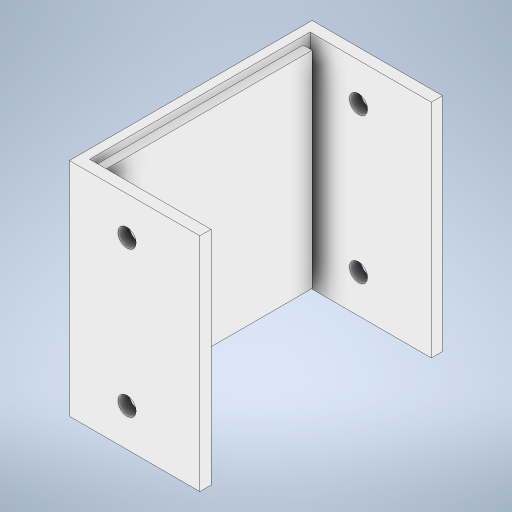
# Autodesk Inventor part: Tapa_R
Saved by Autodesk Inventor 2024 (Build 280153000, 153)
## iProperties
Created: 2023-05-26
Part Number: Tapa_R
Material: Plástico ABS
Document SubType Name: Modeling
Designer: epm01
Density: 1.06 g/cm^3
Appearance: Suave - Blanco
Mass: 7.0225 g
Surface Area: 64.215 cm^2
Volume: 6.625 cm^3
Author: epm01
Autodesk Inventor part; units mm, degrees
ref_plane "YZ Plane" through (0, 0, 0) normal (1, 0, 0) x (0, 1, 0)
ref_plane "XZ Plane" through (0, 0, 0) normal (0, 1, 0) x (-1, 0, 0)
ref_plane "XY Plane" through (0, 0, 0) normal (0, 0, 1) x (1, 0, 0)
sketch "Boceto1" plane through (0, 0, 0) normal (1, 0, 0) x (0, 1, 0)
  line L0 (-17, 17) -> (17, 17)
  line L1 (17, 17) -> (17, -17)
  line L2 (17, -17) -> (-17, -17)
  line L3 (-17, -17) -> (-17, 17)
  line L4 (-17, 17) -> (17, -17) construction
  line L5 (17, 17) -> (-17, -17) construction
  point P0 (0, 0)
  dimension "d0" = 34
  dimension "d1" = 34
  constraints: 12 end point, 2 midpoint, 2 parallel, 1 horizontal, 1 perpendicular
  measures "d0" distance of L0.end L1.end
  measures "d1" distance of L0.start L0.end
extrude "Extrusión1" add sketch "Boceto1" along normal blind 1.5
sketch "Boceto2" plane through (0, 0, 0) normal (-1, 0, 0) x (0, 0, 1)
  line L0 (-20, -18.25) -> (20, -18.25)
  line L1 (20, -18.25) -> (20, 18.25)
  line L2 (20, 18.25) -> (-20, 18.25)
  line L3 (-20, 18.25) -> (-20, -18.25)
  line L4 (-20, -18.25) -> (20, 18.25) construction
  line L5 (20, -18.25) -> (-20, 18.25) construction
  point P0 (0, 0)
  dimension "d4" = 36.5
  dimension "d5" = 40
  constraints: 12 end point, 2 midpoint, 2 parallel, 1 horizontal, 1 perpendicular
  measures "d4" distance of L0.end L1.end
  measures "d5" distance of L1.end L2.end
extrude "Extrusión2" add sketch "Boceto2" along normal blind 1.5
sketch "Boceto3" plane through (0, 0, 0) normal (1, 0, 0) x (0, 0, -1)
  line L0 (-20, 17.8927) -> (-20, -18.25)
  line L1 (-20, 18.25) -> (-20, -18.25)
  line L2 (20, -18.25) -> (-20, -18.25) projected
  line L3 (-18.15, -18.25) -> (-18.15, 18.25)
  line L4 (-18.15, 18.25) -> (-20, 18.25)
  line L5 (-20, -18.25) -> (-18.15, -18.25)
  line L6 (0, 18.25) -> (0, 10.0578) construction
  line L7 (20, 17.8927) -> (20, -18.25)
  line L8 (18.15, -18.25) -> (18.15, 18.25)
  line L9 (18.15, -18.25) -> (20, -18.25)
  point P0 (0, 0)
  dimension "d8" = 1.85
  constraints: 18 end point, 3 symmetric about line, 2 vertical, 1 collinear, 1 horizontal, 1 perpendicular, 1 point on line
  measures "d8" distance between parallel lines of L0 L3
extrude "Extrusión3" add sketch "Boceto3" along normal blind 20
sketch "Boceto4" plane through (0, 0, 0) normal (1, 0, 0) x (0, 0, -1)
  line L0 (20, 18.25) -> (20, -18.25) projected
  line L1 (20, 18.25) -> (20, -18.25)
  line L2 (20, 18.25) -> (18.15, 18.25)
  line L3 (-18.15, 18.25) -> (20, 18.25) projected
  line L4 (18.15, 18.25) -> (18.15, -18.25)
  line L5 (18.15, -18.25) -> (20, -18.25)
  point P0 (0, 0)
  dimension "d11" = 1.85
  constraints: 8 end point, 1 collinear, 1 perpendicular, 1 point on line, 1 vertical
  measures "d11" distance of L0.start L2.end
extrude "Extrusión4" add sketch "Boceto4" along normal blind 20
sketch "Boceto5" plane through (-1.5, -18.25, 20) normal (0, 0, 1) x (1, 0, 0)
  line L0 (1.5, 18.25) -> (9.5, 18.25)
  line L1 (9.5, 18.25) -> (9.5, 30.25)
  line L2 (9.5, 18.25) -> (9.5, 6.25)
  dimension "d14" = 12
  dimension "d15" = 8
  constraints: 6 end point, 1 horizontal, 1 perpendicular, 1 symmetric about line
  measures "d14" distance of L0.end L1.end
  measures "d15" distance of L0.start L0.end
hole "Agujero1" at (8, 12, 20) at (8, -12, 20) direction (0, 0, -1) diameter 3 end through all
